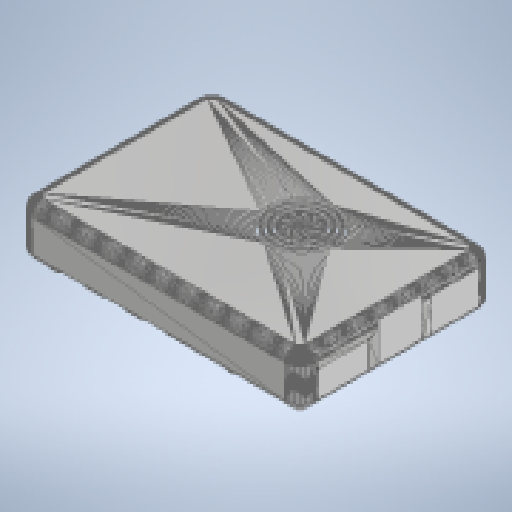
# Autodesk Inventor part: Lid_01
Saved by Autodesk Inventor 2025.2 (Build 292293000, 293)
## iProperties
Created: 2026-02-21
Part Number: Lid_01
Material: 一般
Document SubType Name: Modeling
Designer: naka6
Density: 1 g/cm^3
Appearance: 既定
Author: naka6
Autodesk Inventor part; units mm, degrees
ref_plane "YZ Plane" through (0, 0, 0) normal (1, 0, 0) x (0, 1, 0)
ref_plane "XZ Plane" through (0, 0, 0) normal (0, 1, 0) x (-1, 0, 0)
ref_plane "XY Plane" through (0, 0, 0) normal (0, 0, 1) x (1, 0, 0)
sketch "スケッチ1" plane through (44.5, 6.5, -26.95) normal (0, 0, 1) x (1, 0, 0)
  circle A0 centre (2, 0) radius 0.5 projected
  line L0 (2, 11.003) -> (2, 0.5) projected
  line L1 (-1, 11.0178) -> (-1, -2) projected
  line L2 (-1, -2) -> (-0.0698, -2) projected
  line L3 (0, 0) -> (-0.0698, -2) projected
  line L4 (0, 0) -> (1.5, 0) projected
  line L5 (-1, 11.0178) -> (2, 11.003)
  line L6 (2, 11.42) -> (2, 10.4201) projected
  line L7 (-1, 11.42) -> (2, 11.42)
  line L8 (-1, 11.0178) -> (-1, 11.7705)
  line L9 (-1, 11.42) -> (-1.0338, 11.42)
  point P0 (-44.5, -6.5)
  point P1 (1.5, 0)
  constraints: 8 end point, 2 horizontal, 1 vertical, 1 other
extrude "押し出し1" add sketch "スケッチ1" along normal blind 53.75 contours A0 L4 L3 L2 L1 L5 L0 | L5 L8 L7 L6
sketch "スケッチ2" plane through (43.5, 17.92, -26.95) normal (0, 1, 0) x (1, 0, 0)
  line L0 (3, 0) -> (0, 0) projected
  line L1 (0, 0) -> (0, -53.75) projected
  line L2 (3, -53.75) -> (0, -53.75) projected
  line L3 (3, 0) -> (3, -53.75) projected
  point P0 (-43.5, -26.95)
extrude "押し出し2" add sketch "スケッチ2" along normal blind 2
chamfer "面取り1" distance 0.7 distance2 2 1 edges at (46.5, 19.92, -0.075) measured on face at (46, 19.92, -0.075)
sketch "スケッチ3" plane through (46.4519, 18.4584, 6.05) normal (0, 0, -1) x (-1, 0, 0)
  line L0 (0.6519, 1.4616) -> (2.9519, 1.4616) projected
  line L1 (2.9519, 1.4616) -> (0.6519, 1.4616) projected
  line L2 (-0.0481, -0.5384) -> (0.6519, 1.4616) projected
  line L3 (0.6519, 1.4616) -> (-0.0481, -0.5384) projected
  circle A0 centre (3.4515, -0.5784) radius 3.4996 projected
  line L4 (0.6815, 1.4536) -> (0.6303, 1.4924)
  line L5 (-0.0481, -0.5384) -> (0.6519, 1.4616) projected
  point P0 (46.4519, -18.4584)
  point P1 (0.6559, 1.473)
  point P2 (0.6709, 1.4616)
  point P3 (-0.0479, -0.5377)
  constraints: 2 end point, 1 midpoint, 1 point on line, 2 other
extrude "押し出し3" add sketch "スケッチ3" along normal blind 15.25 contours L2 A0 L4 L0 picked at (0.2131, 0.368)
fillet "フィレット1" radius 0.1 1 edges at (45.8216, 19.9508, -1.575)
